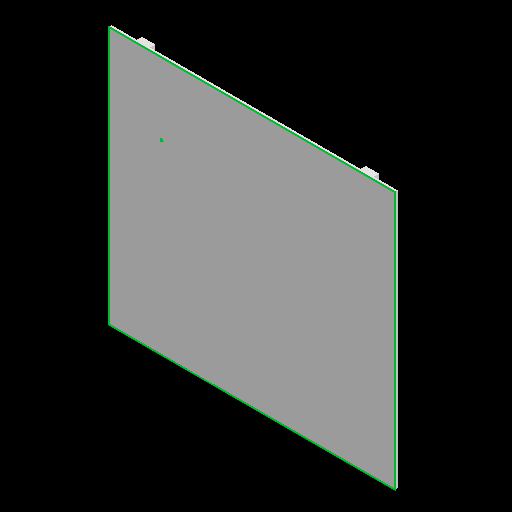
# Autodesk Inventor part: CartTrack
Saved by Autodesk Inventor 2025 (Build 290162000, 162)
## iProperties
Created: 2025-03-15
Part Number: CartTrack
Material: Generic
Document SubType Name: Modeling
Designer: Trevor
Density: 1 g/cm^3
Appearance: Default
Author: Trevor
Autodesk Inventor part; units mm, degrees
ref_plane "YZ Plane" through (0, 0, 0) normal (1, 0, 0) x (0, 1, 0)
ref_plane "XZ Plane" through (0, 0, 0) normal (0, 1, 0) x (-1, 0, 0)
ref_plane "XY Plane" through (0, 0, 0) normal (0, 0, 1) x (1, 0, 0)
sketch "Sketch1" plane through (0, 0, 0) normal (0, 0, 1) x (1, 0, 0)
  line L0 (86.5564, -16.51) -> (86.5564, 16.51) projected
  line L1 (93.1064, -19.05) -> (93.1064, 19.05) projected
  line L2 (86.5564, 19.05) -> (86.5564, -19.05) projected
  line L3 (93.1064, -19.05) -> (93.1064, 19.05) projected
  line L4 (-12.6968, 19.05) -> (-12.6968, -19.05) projected
  line L5 (-6.1468, -19.05) -> (-6.1468, 19.05) projected
  line L6 (-12.6968, -31.75) -> (-12.6968, -69.85) projected
  line L7 (-6.1468, -69.85) -> (-6.1468, -31.75) projected
  line L8 (86.5564, -31.75) -> (86.5564, -69.85) projected
  line L9 (93.1064, -69.85) -> (93.1064, -31.75) projected
  line L10 (-12.6968, -19.05) -> (-12.6968, -31.75)
  line L11 (-6.1468, -31.75) -> (-6.1468, -19.05)
  line L12 (-12.3968, -19.05) -> (-12.3968, 18.85)
  line L13 (-6.4516, 18.85) -> (-6.4516, -19.05)
  line L14 (-6.4516, -19.05) -> (-6.4516, -31.75)
  line L15 (-6.4516, -31.75) -> (-6.4516, -69.65)
  line L16 (-12.3968, -69.65) -> (-12.3968, -31.75)
  line L17 (-12.3968, -31.75) -> (-12.3968, -19.05)
  line L18 (8.247, -25.4) -> (71.6799, -25.4) construction
  line L19 (39.9635, 46.4598) -> (39.9635, -93.3096) construction
  line L20 (-23.5365, 31.75) -> (103.4635, 31.75)
  line L21 (103.4635, 31.75) -> (103.4635, -82.55)
  line L22 (103.4635, -82.55) -> (-23.5365, -82.55)
  line L23 (-23.5365, -82.55) -> (-23.5365, 31.75)
  line L24 (-23.5365, 31.75) -> (103.4635, -82.55) construction
  line L25 (103.4635, 31.75) -> (-23.5365, -82.55) construction
  line L26 (86.5564, -19.05) -> (86.5564, -31.75)
  line L27 (93.1064, -31.75) -> (93.1064, -19.05)
  line L28 (86.5564, 19.05) -> (86.5564, 31.75)
  line L29 (93.1064, 19.05) -> (93.1064, 31.75)
  line L30 (93.1064, -69.85) -> (93.1064, -82.55)
  line L31 (86.5564, -69.85) -> (86.5564, -82.55)
  line L32 (-12.3968, 18.85) -> (-12.3968, 31.75)
  line L33 (-6.4516, 18.85) -> (-6.4516, 31.75)
  line L34 (-6.1468, -69.85) -> (-6.1468, -82.55)
  line L35 (-12.3968, -69.65) -> (-12.3968, -82.55)
  line L36 (-12.6968, 19.05) -> (-12.6968, 31.75)
  line L37 (-6.1468, 19.05) -> (-6.1468, 31.75)
  line L38 (-12.6968, -69.85) -> (-12.6968, -82.55)
  line L39 (-6.4516, -69.65) -> (-6.4516, -82.55)
  line L40 (86.8564, 31.75) -> (86.8564, 19.05)
  line L41 (86.8564, 19.05) -> (86.8564, -19.05)
  line L42 (86.8564, -19.05) -> (86.8564, -31.75)
  line L43 (86.8564, -31.75) -> (86.8564, -69.85)
  line L44 (86.8564, -69.85) -> (86.8564, -82.55)
  line L45 (93.1064, 31.75) -> (93.1064, -82.55)
  line L46 (93.1064, 31.75) -> (93.1064, -82.55)
  line L47 (92.8064, 31.75) -> (92.8064, -82.55)
  point P0 (0, 0)
  point P1 (93.1064, -16.51)
  point P2 (39.9635, -25.4)
  dimension "d0" = 0.3
  dimension "d1" = 127
  dimension "d2" = 114.3
  dimension "d7" = 0.3
  dimension "d8" = 0.3
  dimension "d9" = 0.3048
  constraints: 76 end point, 15 point on line, 11 perpendicular, 6 parallel, 3 collinear, 3 midpoint, 3 vertical, 2 horizontal, 8 other
  measures "d0" distance between parallel lines of L4 L12
  measures "d1" distance of L21.end L22.end
  measures "d2" distance of L20.end L21.end
  measures "d7" distance between parallel lines of L28 L40
  measures "d8" distance between parallel lines of L46 L47
  measures "d9" distance between parallel lines of L5 L13
extrude "Extrusion1" add sketch "Sketch1" against normal blind 2.286 contours L20 L47 L22 L44 L43 L42 L41 L40 | L33 L13 L14 L15 L39 L22 L35 L16 L17 L12 L32 L20
sketch "Sketch2" plane through (0, 0, 0) normal (0, 0, 1) x (1, 0, 0)
  line L0 (103.4635, 31.75) -> (103.4635, -82.55) projected
  line L1 (-23.5365, 31.75) -> (103.4635, 31.75) projected
  line L2 (-23.5365, -82.55) -> (-23.5365, 31.75) projected
  line L3 (103.4635, -82.55) -> (-23.5365, -82.55) projected
  point P0 (0, 0)
  point P1 (93.1064, 31.75)
extrude "Extrusion2" add sketch "Sketch2" along normal blind 1.27
sketch "Sketch3" plane through (0, 0, 1.27) normal (0, 0, 1) x (1, 0, 0)
  line L0 (-23.5365, 31.75) -> (-23.5365, -82.55) projected
  line L1 (-23.5365, -82.55) -> (103.4635, -82.55) projected
  line L2 (103.4635, -82.55) -> (103.4635, 31.75) projected
  line L3 (103.4635, 31.75) -> (-23.5365, 31.75) projected
  point P0 (0, 0)
body "Solid1"
